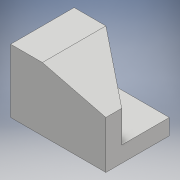
# Autodesk Inventor part: 50
Saved by Autodesk Inventor 2017 (Build 210142000, 142)
## iProperties
Part Number: 50
Material: 一般
Document SubType Name: Modeling
Designer: Brian
Density: 1 g/cm^3
Appearance: 預設
Author: Brian
Autodesk Inventor part; units mm, degrees
ref_plane "YZ Plane" through (0, 0, 0) normal (1, 0, 0) x (0, 1, 0)
ref_plane "XZ Plane" through (0, 0, 0) normal (0, 1, 0) x (-1, 0, 0)
ref_plane "XY Plane" through (0, 0, 0) normal (0, 0, 1) x (1, 0, 0)
sketch "草圖1" plane through (0, 0, 0) normal (0, 1, 0) x (-1, 0, 0)
  line L0 (0, 0) -> (-60, 0)
  line L1 (-60, 0) -> (-60, -40)
  line L2 (-60, -40) -> (0, -40)
  line L3 (0, -40) -> (0, 0)
  dimension "d0" = 40
  dimension "d1" = 60
  constraints: 8 end point, 2 parallel, 1 horizontal, 1 perpendicular
  measures "d0" distance of L2.end L0.start
  measures "d1" distance of L1.end L2.end
extrude "擠出1" add sketch "草圖1" along normal blind 40
sketch "草圖2" plane through (0, 40, 0) normal (0, 1, 0) x (1, 0, 0)
  line L0 (60, 0) -> (60, 40) projected
  line L1 (60, 10) -> (20, 0)
  line L2 (0, 0) -> (60, 0) projected
  dimension "d4" = 10
  dimension "d5" = 40
  constraints: 2 end point, 1 point on line
  measures "d4" vertical distance of L1.start L1.end
  measures "d5" horizontal distance of L1.start L1.end
extrude "擠出2" cut sketch "草圖2" against normal through all fills toward (40.0121, 4.9515) open curves L1
sketch "草圖3" plane through (0, 0, 0) normal (0, 0, 1) x (1, 0, 0)
  line L0 (20, 0) -> (20, 40) projected
  line L1 (20, 40) -> (60, 10)
  line L2 (60, 10) -> (83.2965, 35.9899)
  line L3 (83.2965, 35.9899) -> (54.3256, 64.0339)
  line L4 (20, 40) -> (60, 40) projected
  line L5 (54.3256, 64.0339) -> (20, 40)
  point P0 (0, 0)
  dimension "d9" = 30
  dimension "d10" = 40
  constraints: 8 end point
  measures "d9" vertical distance of L0.end L1.end
  measures "d10" horizontal distance of L0.end L1.end
extrude "擠出3" cut sketch "草圖3" against normal blind 30
